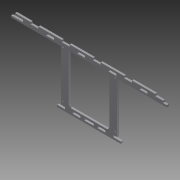
# Autodesk Inventor part: back
Saved by Autodesk Inventor 2011 (Build 150239000, 239)
## iProperties
Created: 2011-08-21
Part Number: back
Document SubType Name: Modeling
Designer: Matthew
Density: 1 g/cm^3
Author: Matthew
Autodesk Inventor part; units mm, degrees
ref_plane "YZ Plane" through (0, 0, 0) normal (1, 0, 0) x (0, 1, 0)
ref_plane "XZ Plane" through (0, 0, 0) normal (0, 1, 0) x (-1, 0, 0)
ref_plane "XY Plane" through (0, 0, 0) normal (0, 0, 1) x (1, 0, 0)
sketch "Sketch1" plane through (0, 0, 0) normal (0, 0, 1) x (1, 0, 0)
  line L0 (-267.7504, 67.4597) -> (240.2496, 67.4597)
  line L1 (240.2496, 67.4597) -> (240.2496, -986.6403)
  line L2 (240.2496, -986.6403) -> (-267.7504, -986.6403)
  line L3 (-267.7504, -986.6403) -> (-267.7504, 67.4597)
  point P0 (0, 0)
  dimension "d0" = 508
  dimension "d1" = 1054.1
  constraints: 8 end point, 2 parallel, 1 horizontal, 1 perpendicular
  measures "d0" distance of L1.end L2.end
  measures "d1" distance of L0.end L1.end
extrude "Extrusion1" add sketch "Sketch1" along normal blind 6.35
sketch "Sketch2" plane through (0, 0, 6.35) normal (0, 0, 1) x (1, 0, 0)
  line L0 (240.2496, -986.6403) -> (-267.7504, -986.6403) projected
  line L1 (-267.7504, -986.6403) -> (-13.7504, -986.6403)
  line L2 (-13.7504, -986.6403) -> (-13.7504, -980.2903)
  line L3 (-13.7504, -980.2903) -> (1.4896, -980.2903)
  line L4 (1.4896, -980.2903) -> (-28.9904, -980.2903)
  line L5 (-28.9904, -980.2903) -> (1.4896, -980.2903)
  line L6 (1.4896, -980.2903) -> (1.4896, -973.9403)
  line L7 (1.4896, -973.9403) -> (-28.9904, -973.9403)
  line L8 (-28.9904, -973.9403) -> (-28.9904, -980.2903)
  point P0 (0, 0)
  dimension "d4" = 254
  dimension "d5" = 6.35
  dimension "d6" = 15.24
  dimension "d7" = 30.48
  dimension "d8" = 6.35
  constraints: 16 end point, 4 parallel, 2 perpendicular, 1 horizontal, 1 midpoint
  measures "d4" distance of L0.end L1.end
  measures "d5" distance of L1.end L2.end
  measures "d6" distance of L2.end L3.end
  measures "d7" distance of L3.end L4.end
  measures "d8" distance of L6.end L5.end
extrude "Extrusion2" cut sketch "Sketch2" against normal blind 104.14
sketch "Sketch3" plane through (0, 0, 6.35) normal (0, 0, 1) x (1, 0, 0)
  line L0 (240.2496, -986.6403) -> (-267.7504, -986.6403) projected
  line L1 (1.4896, -980.2903) -> (14.1896, -980.2903)
  line L2 (-28.9904, -980.2903) -> (-41.6904, -980.2903)
  line L3 (-41.6904, -980.2903) -> (-67.0904, -980.2903)
  line L4 (-67.0904, -980.2903) -> (-67.0904, -973.9403)
  line L5 (-67.0904, -973.9403) -> (-41.6904, -973.9403)
  line L6 (-41.6904, -973.9403) -> (-41.6904, -980.2903)
  line L7 (14.1896, -980.2903) -> (39.5896, -980.2903)
  line L8 (39.5896, -980.2903) -> (39.5896, -973.9403)
  line L9 (39.5896, -973.9403) -> (14.1896, -973.9403)
  line L10 (14.1896, -973.9403) -> (14.1896, -980.2903)
  point P0 (0, 0)
  dimension "d11" = 12.7
  dimension "d12" = 12.7
  dimension "d13" = 25.4
  dimension "d14" = 25.4
  constraints: 20 end point, 5 parallel, 2 horizontal, 2 perpendicular, 1 collinear
  measures "d11" distance of L1.start L1.end
  measures "d12" distance of L2.start L2.end
  measures "d13" distance of L4.end L5.end
  measures "d14" distance of L9.end L8.end
extrude "Extrusion3" cut sketch "Sketch3" against normal blind 104.14
sketch "Sketch4" plane through (0, 0, 6.35) normal (0, 0, 1) x (1, 0, 0)
  line L0 (-67.0904, -973.9403) -> (-41.6904, -973.9403) projected
  line L1 (14.1896, -973.9403) -> (39.5896, -973.9403) projected
  line L2 (-28.9904, -973.9403) -> (1.4896, -973.9403) projected
  line L3 (240.2496, 67.4597) -> (240.2496, -986.6403) projected
  line L4 (-267.7504, -986.6403) -> (-267.7504, 67.4597) projected
  line L5 (240.2496, -986.6403) -> (-267.7504, -986.6403) projected
  line L6 (-67.0904, -980.2903) -> (-92.4904, -980.2903)
  line L7 (-92.4904, -980.2903) -> (-117.8904, -980.2903)
  line L8 (-117.8904, -980.2903) -> (-117.8904, -986.6403)
  line L9 (39.5896, -980.2903) -> (64.9896, -980.2903)
  line L10 (64.9896, -980.2903) -> (90.3896, -980.2903)
  line L11 (90.3896, -980.2903) -> (90.3896, -986.6403)
  line L12 (-41.6904, -973.9403) -> (-28.9904, -973.9403)
  line L13 (1.4896, -973.9403) -> (14.1896, -973.9403)
  line L14 (-67.0904, -973.9403) -> (-79.7904, -973.9403)
  line L15 (39.5896, -973.9403) -> (52.2896, -973.9403)
  line L16 (-79.7904, -973.9403) -> (-79.7904, -802.4903)
  line L17 (52.2896, -973.9403) -> (52.2896, -802.4903)
  line L18 (52.2896, -802.4903) -> (-79.7904, -802.4903)
  line L19 (-79.7904, -802.4903) -> (-105.1904, -802.4903)
  line L20 (-105.1904, -802.4903) -> (-105.1904, -815.1903)
  line L21 (-105.1904, -815.1903) -> (-92.4904, -815.1903)
  line L22 (-92.4904, -815.1903) -> (-92.4904, -980.2903)
  line L23 (64.9896, -980.2903) -> (64.9896, -815.1903)
  line L24 (64.9896, -815.1903) -> (77.6896, -815.1903)
  line L25 (77.6896, -815.1903) -> (77.6896, -802.4903)
  line L26 (77.6896, -802.4903) -> (52.2896, -802.4903)
  line L27 (-105.1904, -802.4903) -> (-267.7504, -802.4903)
  line L28 (77.6896, -802.4903) -> (240.2496, -802.4903)
  point P0 (0, 0)
  dimension "d17" = 25.4
  dimension "d18" = 25.4
  dimension "d19" = 25.4
  dimension "d20" = 25.4
  dimension "d21" = 171.45
  dimension "d22" = 25.4
  dimension "d23" = 12.7
  constraints: 46 end point, 10 perpendicular, 8 parallel, 5 collinear, 4 point on line
  measures "d17" distance of L6.start L6.end
  measures "d18" distance of L6.end L7.end
  measures "d19" distance of L9.start L9.end
  measures "d20" distance of L9.end L10.end
  measures "d21" distance of L14.end L16.end
  measures "d22" distance of L16.end L19.end
  measures "d23" distance of L19.end L20.end
extrude "Extrusion4" cut sketch "Sketch4" against normal blind 104.14 contours L14 L16 L18 L17 L15 L1 L13 L2 L12 L0 | L20 L21 L22 L7 L8 L5 L4 L27 | L28 L3 L5 L11 L10 L23 L24 L25
sketch "Sketch5" plane through (0, 0, 6.35) normal (0, 0, 1) x (1, 0, 0)
  line L0 (-92.4904, -815.1903) -> (-92.4904, -980.2903) projected
  line L1 (64.9896, -980.2903) -> (64.9896, -815.1903) projected
  line L2 (-92.4904, -973.9403) -> (-92.4904, -967.5903)
  line L3 (-92.4904, -967.5903) -> (-105.1904, -967.5903)
  line L4 (-105.1904, -967.5903) -> (-105.1904, -954.8903)
  line L5 (-105.1904, -954.8903) -> (-92.4904, -954.8903)
  line L6 (64.9896, -954.8903) -> (77.6896, -954.8903)
  line L7 (77.6896, -954.8903) -> (77.6896, -967.5903)
  line L8 (77.6896, -967.5903) -> (64.9896, -967.5903)
  point P0 (0, 0)
  dimension "d26" = 6.35
  dimension "d27" = 12.7
  constraints: 14 end point, 5 point on line, 3 perpendicular, 2 parallel, 1 collinear
  measures "d26" distance of L2.start L2.end
  measures "d27" distance of L3.end L4.end
extrude "Extrusion5" add sketch "Sketch5" against normal blind 6.35
sketch "Sketch6" plane through (0, 0, 6.35) normal (0, 0, 1) x (1, 0, 0)
  line L0 (-79.7904, -802.4903) -> (52.2896, -802.4903) projected
  line L1 (-267.7504, -802.4903) -> (-105.1904, -802.4903) projected
  line L2 (77.6896, -802.4903) -> (240.2496, -802.4903) projected
  line L3 (-267.7504, -802.4903) -> (-242.3504, -802.4903)
  line L4 (-242.3504, -802.4903) -> (-216.9504, -802.4903)
  line L5 (-216.9504, -802.4903) -> (-140.7504, -802.4903)
  line L6 (-140.7504, -802.4903) -> (-115.3504, -802.4903)
  line L7 (-115.3504, -802.4903) -> (-39.1504, -802.4903)
  line L8 (-39.1504, -802.4903) -> (-13.7504, -802.4903)
  line L9 (-13.7504, -802.4903) -> (62.4496, -802.4903)
  line L10 (62.4496, -802.4903) -> (87.8496, -802.4903)
  line L11 (87.8496, -802.4903) -> (164.0496, -802.4903)
  line L12 (164.0496, -802.4903) -> (189.4496, -802.4903)
  line L13 (189.4496, -802.4903) -> (265.6496, -802.4903)
  line L14 (265.6496, -802.4903) -> (240.2496, -802.4903)
  line L15 (-242.3504, -802.4903) -> (-216.9504, -802.4903)
  line L16 (-216.9504, -802.4903) -> (-216.9504, -796.1403)
  line L17 (-216.9504, -796.1403) -> (-242.3504, -796.1403)
  line L18 (-242.3504, -796.1403) -> (-242.3504, -802.4903)
  line L19 (-140.7504, -802.4903) -> (-115.3504, -802.4903)
  line L20 (-115.3504, -802.4903) -> (-115.3504, -796.1403)
  line L21 (-115.3504, -796.1403) -> (-140.7504, -796.1403)
  line L22 (-140.7504, -796.1403) -> (-140.7504, -802.4903)
  line L23 (-39.1504, -802.4903) -> (-13.7504, -802.4903)
  line L24 (-13.7504, -802.4903) -> (-13.7504, -796.1403)
  line L25 (-13.7504, -796.1403) -> (-39.1504, -796.1403)
  line L26 (-39.1504, -796.1403) -> (-39.1504, -802.4903)
  line L27 (62.4496, -802.4903) -> (87.8496, -802.4903)
  line L28 (87.8496, -802.4903) -> (87.8496, -796.1403)
  line L29 (87.8496, -796.1403) -> (62.4496, -796.1403)
  line L30 (62.4496, -796.1403) -> (62.4496, -802.4903)
  line L31 (164.0496, -802.4903) -> (189.4496, -802.4903)
  line L32 (189.4496, -802.4903) -> (189.4496, -796.1403)
  line L33 (189.4496, -796.1403) -> (164.0496, -796.1403)
  line L34 (164.0496, -796.1403) -> (164.0496, -802.4903)
  point P0 (0, 0)
  dimension "d30" = 25.4
  dimension "d31" = 25.4
  dimension "d32" = 76.2
  dimension "d33" = 25.4
  dimension "d34" = 76.2
  dimension "d35" = 25.4
  dimension "d36" = 76.2
  dimension "d37" = 25.4
  dimension "d38" = 76.2
  dimension "d39" = 25.4
  dimension "d40" = 76.2
  dimension "d41" = 25.4
  dimension "d42" = 6.35
  constraints: 64 end point, 10 parallel, 10 point on line, 5 horizontal, 5 perpendicular, 1 collinear, 1 midpoint
  measures "d30" distance of L1.start L3.end
  measures "d31" distance of L3.end L4.end
  measures "d32" distance of L4.end L5.end
  measures "d33" distance of L5.end L6.end
  measures "d34" distance of L6.end L7.end
  measures "d35" distance of L7.end L8.end
  measures "d36" distance of L8.end L9.end
  measures "d37" distance of L9.end L10.end
  measures "d38" distance of L10.end L11.end
  measures "d39" distance of L11.end L12.end
  measures "d40" distance of L12.end L13.end
  measures "d41" distance of L13.end L2.end
  measures "d42" distance of L16.end L15.end
extrude "Extrusion6" cut sketch "Sketch6" against normal blind 25.4
sketch "Sketch7" plane through (0, 0, 6.35) normal (0, 0, 1) x (1, 0, 0)
  line L0 (-267.7504, -802.4903) -> (240.2496, -802.4903)
  line L1 (240.2496, -802.4903) -> (240.2496, -808.8403)
  line L2 (240.2496, -808.8403) -> (-267.7504, -808.8403)
  line L3 (-267.7504, -808.8403) -> (-267.7504, -802.4903)
  point P0 (0, 0)
  constraints: 8 end point, 2 parallel, 1 horizontal, 1 perpendicular
extrude "Extrusion7" add sketch "Sketch7" against normal blind 6.35
sketch "Sketch8" plane through (0, 0, 6.35) normal (0, 0, 1) x (1, 0, 0)
  line L0 (-216.9504, -796.1403) -> (-191.5504, -796.1403)
  line L1 (-191.5504, -796.1403) -> (-191.5504, -789.7903)
  line L2 (-191.5504, -789.7903) -> (-216.9504, -789.7903)
  line L3 (-216.9504, -789.7903) -> (-216.9504, -796.1403)
  line L4 (-115.3504, -796.1403) -> (-89.9504, -796.1403)
  line L5 (-89.9504, -796.1403) -> (-89.9504, -789.7903)
  line L6 (-89.9504, -789.7903) -> (-115.3504, -789.7903)
  line L7 (-115.3504, -789.7903) -> (-115.3504, -796.1403)
  line L8 (-13.7504, -796.1403) -> (11.6496, -796.1403)
  line L9 (11.6496, -796.1403) -> (11.6496, -789.7903)
  line L10 (11.6496, -789.7903) -> (-13.7504, -789.7903)
  line L11 (-13.7504, -789.7903) -> (-13.7504, -796.1403)
  line L12 (87.8496, -796.1403) -> (113.2496, -796.1403)
  line L13 (113.2496, -796.1403) -> (113.2496, -789.7903)
  line L14 (113.2496, -789.7903) -> (87.8496, -789.7903)
  line L15 (87.8496, -789.7903) -> (87.8496, -796.1403)
  line L16 (189.4496, -796.1403) -> (214.8496, -796.1403)
  line L17 (214.8496, -796.1403) -> (214.8496, -789.7903)
  line L18 (214.8496, -789.7903) -> (189.4496, -789.7903)
  line L19 (189.4496, -789.7903) -> (189.4496, -796.1403)
  point P0 (0, 0)
  dimension "d47" = 25.4
  dimension "d48" = 6.35
  dimension "d49" = 25.4
  dimension "d50" = 25.4
  dimension "d51" = 25.4
  dimension "d52" = 25.4
  constraints: 40 end point, 10 parallel, 5 horizontal, 5 perpendicular
  measures "d47" distance of L2.end L1.end
  measures "d48" distance of L1.end L0.end
  measures "d49" distance of L6.end L5.end
  measures "d50" distance of L10.end L9.end
  measures "d51" distance of L14.end L13.end
  measures "d52" distance of L18.end L17.end
extrude "Extrusion8" cut sketch "Sketch8" against normal blind 6.35
sketch "Sketch9" plane through (0, 0, 6.35) normal (0, 0, 1) x (1, 0, 0)
  circle A0 centre (-98.8404, -808.8403) radius 1.9812
  circle A1 centre (-98.8404, -961.2403) radius 1.9812
  circle A2 centre (71.3396, -961.2403) radius 1.9812
  circle A3 centre (71.3396, -808.8403) radius 1.9812
  point P0 (0, 0)
  dimension "d55" = 3.9624
  dimension "d56" = 3.9624
  dimension "d57" = 3.9624
  dimension "d58" = 3.9624
  constraints: 4 centre point
  measures "d55" diameter of A0
  measures "d56" diameter of A1
  measures "d57" diameter of A2
  measures "d58" diameter of A3
extrude "Extrusion9" cut sketch "Sketch9" against normal blind 6.35
sketch "Sketch10" plane through (0, 0, 0) normal (0, 0, -1) x (-1, 0, 0)
  line L0 (-77.6896, -815.1903) -> (-64.9896, -815.1903) projected
  line L1 (-64.9896, -815.1903) -> (-64.9896, -954.8903) projected
  line L2 (-77.6896, -954.8903) -> (-64.9896, -954.8903) projected
  line L3 (-64.9896, -967.5903) -> (-77.6896, -967.5903) projected
  line L4 (-64.9896, -967.5903) -> (-64.9896, -980.2903) projected
  line L5 (92.4904, -980.2903) -> (92.4904, -967.5903) projected
  line L6 (105.1904, -967.5903) -> (92.4904, -967.5903) projected
  line L7 (92.4904, -954.8903) -> (105.1904, -954.8903) projected
  line L8 (92.4904, -954.8903) -> (92.4904, -815.1903) projected
  line L9 (92.4904, -815.1903) -> (105.1904, -815.1903) projected
  line L10 (-77.6896, -808.8403) -> (-240.2496, -808.8403) projected
  line L11 (-77.6896, -815.1903) -> (-77.6896, -954.8903)
  line L12 (105.1904, -954.8903) -> (105.1904, -815.1903)
  line L13 (105.1904, -967.5903) -> (105.1904, -973.9403)
  line L14 (105.1904, -973.9403) -> (92.4904, -973.9403)
  line L15 (-77.6896, -967.5903) -> (-77.6896, -973.9403)
  line L16 (-77.6896, -973.9403) -> (-64.9896, -973.9403)
  point P0 (0, 0)
  constraints: 12 end point, 2 midpoint, 2 perpendicular, 1 collinear, 1 parallel
extrude "Extrusion10" add sketch "Sketch10" against normal blind 6.35
sketch "Sketch11" plane through (0, 0, 0) normal (0, 0, -1) x (-1, 0, 0)
  line L0 (79.7904, -808.8403) -> (79.7904, -973.9403) projected
  line L1 (79.7904, -973.9403) -> (67.0904, -973.9403) projected
  line L2 (-39.5896, -973.9403) -> (-52.2896, -973.9403) projected
  line L3 (-52.2896, -973.9403) -> (-52.2896, -808.8403) projected
  line L4 (-39.5896, -973.9403) -> (-52.2896, -961.2403)
  line L5 (67.0904, -973.9403) -> (79.7904, -961.2403)
  line L6 (-45.9396, -967.5903) -> (73.4404, -967.5903)
  line L7 (-39.5896, -973.9403) -> (67.0904, -973.9403)
  point P0 (0, 0)
  constraints: 8 end point, 2 midpoint, 2 point on line, 1 perpendicular
extrude "Extrusion11" add sketch "Sketch11" against normal blind 6.35
sketch "Sketch12" plane through (0, 0, 0) normal (0, 0, -1) x (-1, 0, 0)
  line L0 (267.7504, -808.8403) -> (267.7504, 67.4597) projected
  line L1 (-240.2496, 67.4597) -> (-240.2496, -808.8403) projected
  line L2 (-240.2496, 67.4597) -> (-214.8496, 67.4597)
  line L3 (-214.8496, 67.4597) -> (-214.8496, 42.0597)
  line L4 (-214.8496, 42.0597) -> (-240.2496, 42.0597)
  line L5 (-240.2496, 42.0597) -> (-240.2496, 67.4597)
  line L6 (267.7504, 67.4597) -> (242.3504, 67.4597)
  line L7 (242.3504, 67.4597) -> (242.3504, 42.0597)
  line L8 (242.3504, 42.0597) -> (267.7504, 42.0597)
  line L9 (267.7504, 42.0597) -> (267.7504, 67.4597)
  line L10 (-240.2496, -789.7903) -> (-214.8496, -789.7903)
  line L11 (-214.8496, -789.7903) -> (-214.8496, -764.3903)
  line L12 (-214.8496, -764.3903) -> (-240.2496, -764.3903)
  line L13 (-240.2496, -764.3903) -> (-240.2496, -789.7903)
  line L14 (267.7504, -789.7903) -> (242.3504, -789.7903)
  line L15 (242.3504, -789.7903) -> (242.3504, -764.3903)
  line L16 (242.3504, -764.3903) -> (267.7504, -764.3903)
  line L17 (267.7504, -764.3903) -> (267.7504, -789.7903)
  line L18 (-214.8496, -764.3903) -> (242.3504, -764.3903)
  line L19 (242.3504, -764.3903) -> (242.3504, 42.0597)
  line L20 (242.3504, 42.0597) -> (-214.8496, 42.0597)
  line L21 (-214.8496, 42.0597) -> (-214.8496, -764.3903)
  point P0 (0, 0)
  dimension "d65" = 25.4
  dimension "d66" = 25.4
  dimension "d67" = 25.4
  dimension "d68" = 25.4
  dimension "d69" = 25.4
  dimension "d70" = 25.4
  dimension "d71" = 25.4
  dimension "d72" = 25.4
  constraints: 40 end point, 10 parallel, 5 horizontal, 5 perpendicular, 2 point on line
  measures "d65" distance of L3.end L4.end
  measures "d66" distance of L2.end L3.end
  measures "d67" distance of L8.end L7.end
  measures "d68" distance of L7.end L6.end
  measures "d69" distance of L12.end L11.end
  measures "d70" distance of L11.end L10.end
  measures "d71" distance of L15.end L16.end
  measures "d72" distance of L14.end L15.end
extrude "Extrusion12" cut sketch "Sketch12" against normal blind 6.35 contours L18 L21 L20 L19
fillet "Fillet1" radius 12.7 1 edges at (-242.3504, 42.0597, 3.175)
fillet "Fillet2" radius 12.7 3 edges at (214.8496, 42.0597, 3.175) (214.8496, -764.3903, 3.175) (-242.3504, -764.3903, 3.175)
sketch "Sketch13" plane through (0, 0, 0) normal (0, 0, -1) x (-1, 0, 0)
  line L0 (-214.8496, -751.6903) -> (-214.8496, 29.3597) projected
  arc A0 (-202.1496, 42.0597) -> (-214.8496, 29.3597) centre (-202.1496, 29.3597) ccw projected
  line L1 (-202.1496, 42.0597) -> (229.6504, 42.0597) projected
  arc A1 (242.3504, 29.3597) -> (229.6504, 42.0597) centre (229.6504, 29.3597) ccw projected
  line L2 (242.3504, 29.3597) -> (242.3504, -751.6903) projected
  arc A2 (229.6504, -764.3903) -> (242.3504, -751.6903) centre (229.6504, -751.6903) ccw projected
  arc A3 (-214.8496, -751.6903) -> (-202.1496, -764.3903) centre (-202.1496, -751.6903) ccw projected
  line L3 (267.7504, -808.8403) -> (267.7504, 67.4597) projected
  line L4 (267.7504, 67.4597) -> (-240.2496, 67.4597) projected
  line L5 (-240.2496, 67.4597) -> (-240.2496, -808.8403) projected
  line L6 (-202.1496, -764.3903) -> (-240.2496, -764.3903)
  line L7 (229.6504, -764.3903) -> (267.7504, -764.3903)
  point P0 (0, 0)
  constraints: 4 end point, 2 perpendicular, 2 point on line, 2 tangent
extrude "Extrusion13" cut sketch "Sketch13" against normal blind 25.4
sketch "Sketch14" plane through (0, 0, 0) normal (0, 0, -1) x (-1, 0, 0)
  line L0 (-240.2496, -764.3903) -> (-202.1496, -764.3903)
  line L1 (-202.1496, -764.3903) -> (-202.1496, -688.1903)
  line L2 (-202.1496, -688.1903) -> (-240.2496, -688.1903)
  line L3 (-240.2496, -688.1903) -> (-240.2496, -764.3903)
  line L4 (267.7504, -764.3903) -> (229.6504, -764.3903)
  line L5 (229.6504, -764.3903) -> (229.6504, -688.1903)
  line L6 (229.6504, -688.1903) -> (267.7504, -688.1903)
  line L7 (267.7504, -688.1903) -> (267.7504, -764.3903)
  point P0 (0, 0)
  dimension "d79" = 76.2
  dimension "d80" = 76.2
  constraints: 16 end point, 4 parallel, 2 horizontal, 2 perpendicular
  measures "d79" distance of L1.end L0.end
  measures "d80" distance of L4.end L5.end
extrude "Extrusion14" add sketch "Sketch14" against normal blind 6.35
sketch "Sketch15" plane through (0, 0, 0) normal (0, 0, -1) x (-1, 0, 0)
  line L0 (-240.2496, -688.1903) -> (-221.1996, -688.1903)
  line L1 (-221.1996, -688.1903) -> (-221.1996, -707.2403)
  line L2 (-221.1996, -707.2403) -> (-240.2496, -707.2403)
  line L3 (-240.2496, -707.2403) -> (-240.2496, -688.1903)
  line L4 (267.7504, -688.1903) -> (248.7004, -688.1903)
  line L5 (248.7004, -688.1903) -> (248.7004, -707.2403)
  line L6 (248.7004, -707.2403) -> (267.7504, -707.2403)
  line L7 (267.7504, -707.2403) -> (267.7504, -688.1903)
  circle A0 centre (248.7004, -707.2403) radius 1.9812
  circle A1 centre (-221.1996, -707.2403) radius 1.9812
  point P0 (0, 0)
  dimension "d83" = 19.05
  dimension "d84" = 19.05
  dimension "d85" = 19.05
  dimension "d86" = 19.05
  dimension "d87" = 3.9624
  dimension "d88" = 3.9624
  constraints: 16 end point, 4 parallel, 2 centre point, 2 coincident, 2 horizontal, 2 perpendicular
  measures "d83" distance of L1.end L2.end
  measures "d84" distance of L0.end L1.end
  measures "d85" distance of L6.end L5.end
  measures "d86" distance of L5.end L4.end
  measures "d87" diameter of A0
  measures "d88" diameter of A1
extrude "Extrusion15" cut sketch "Sketch15" against normal blind 6.35 contours A1 L2 L1 | L1 L2 A1 | A0 L6 L5 | L5 L6 A0
sketch "Sketch16" plane through (0, 0, 0) normal (0, 0, -1) x (-1, 0, 0)
  line L0 (-240.2496, -688.1903) -> (-240.2496, -808.8403) projected
  line L1 (-240.2496, -688.1903) -> (-233.8996, -688.1903)
  line L2 (-233.8996, -688.1903) -> (-233.8996, -713.5903)
  line L3 (-233.8996, -713.5903) -> (-240.2496, -713.5903)
  line L4 (-240.2496, -713.5903) -> (-240.2496, -688.1903)
  line L5 (-233.8996, -713.5903) -> (-240.2496, -713.5903)
  line L6 (-240.2496, -713.5903) -> (-240.2496, -738.9903)
  line L7 (-240.2496, -738.9903) -> (-233.8996, -738.9903)
  line L8 (-233.8996, -738.9903) -> (-233.8996, -713.5903)
  line L9 (-233.8996, -738.9903) -> (-240.2496, -738.9903)
  line L10 (-240.2496, -738.9903) -> (-240.2496, -764.3903)
  line L11 (-240.2496, -764.3903) -> (-233.8996, -764.3903)
  line L12 (-233.8996, -764.3903) -> (-233.8996, -738.9903)
  line L13 (-233.8996, -764.3903) -> (-240.2496, -764.3903)
  line L14 (-240.2496, -764.3903) -> (-240.2496, -789.7903)
  line L15 (-240.2496, -789.7903) -> (-233.8996, -789.7903)
  line L16 (-233.8996, -789.7903) -> (-233.8996, -764.3903)
  point P0 (0, 0)
  dimension "d91" = 6.35
  dimension "d92" = 25.4
  dimension "d93" = 25.4
  dimension "d94" = 25.4
  constraints: 32 end point, 8 parallel, 4 horizontal, 4 perpendicular, 3 point on line
  measures "d91" distance of L2.end L3.end
  measures "d92" distance of L1.end L2.end
  measures "d93" distance of L6.end L5.end
  measures "d94" distance of L10.end L9.end
extrude "Extrusion16" cut sketch "Sketch16" against normal blind 6.35 contours L1 L2 L3 L0 | L7 L12 L11 L0
sketch "Sketch17" plane through (0, 0, 0) normal (0, 0, -1) x (-1, 0, 0)
  line L0 (267.7504, -808.8403) -> (267.7504, -688.1903) projected
  line L1 (267.7504, -688.1903) -> (261.4004, -688.1903)
  line L2 (261.4004, -688.1903) -> (261.4004, -713.5903)
  line L3 (261.4004, -713.5903) -> (267.7504, -713.5903)
  line L4 (267.7504, -713.5903) -> (267.7504, -688.1903)
  line L5 (261.4004, -713.5903) -> (267.7504, -713.5903)
  line L6 (267.7504, -713.5903) -> (267.7504, -738.9903)
  line L7 (267.7504, -738.9903) -> (261.4004, -738.9903)
  line L8 (261.4004, -738.9903) -> (261.4004, -713.5903)
  line L9 (261.4004, -738.9903) -> (267.7504, -738.9903)
  line L10 (267.7504, -738.9903) -> (267.7504, -764.3903)
  line L11 (267.7504, -764.3903) -> (261.4004, -764.3903)
  line L12 (261.4004, -764.3903) -> (261.4004, -738.9903)
  point P0 (0, 0)
  dimension "d97" = 6.35
  dimension "d98" = 25.4
  dimension "d99" = 25.4
  dimension "d100" = 25.4
  constraints: 24 end point, 6 parallel, 3 horizontal, 3 perpendicular, 2 point on line
  measures "d97" distance of L3.end L2.end
  measures "d98" distance of L2.end L1.end
  measures "d99" distance of L5.end L6.end
  measures "d100" distance of L9.end L10.end
extrude "Extrusion17" cut sketch "Sketch17" against normal blind 6.35 contours L11 L12 L7 L0 | L3 L2 L1 L0
sketch "Sketch18" plane through (0, 0, 0) normal (0, 0, -1) x (-1, 0, 0)
  circle A0 centre (-221.1996, -707.2403) radius 1.9812 projected
  circle A1 centre (248.7004, -707.2403) radius 1.9812 projected
  line L0 (-233.8996, -688.1903) -> (261.4004, -688.1903)
  line L1 (261.4004, -688.1903) -> (261.4004, -713.5903)
  line L2 (261.4004, -713.5903) -> (-233.8996, -713.5903)
  line L3 (-233.8996, -713.5903) -> (-233.8996, -688.1903)
  point P0 (0, 0)
  constraints: 8 end point, 2 parallel, 1 horizontal, 1 perpendicular
extrude "Extrusion18" cut sketch "Sketch18" against normal blind 25.4
sketch "Sketch19" plane through (0, 0, 0) normal (0, 0, -1) x (-1, 0, 0)
  line L0 (-202.1496, -713.5903) -> (-221.1996, -713.5903)
  line L1 (-221.1996, -713.5903) -> (-221.1996, -726.2903)
  line L2 (-221.1996, -726.2903) -> (-202.1496, -726.2903)
  line L3 (-202.1496, -726.2903) -> (-202.1496, -713.5903)
  circle A0 centre (-221.1996, -726.2903) radius 1.9812
  circle A1 centre (248.7004, -728.2715) radius 1.9812
  point P0 (0, 0)
  dimension "d105" = 19.05
  dimension "d106" = 12.7
  dimension "d107" = 3.9624
  dimension "d108" = 3.9624
  constraints: 8 end point, 2 centre point, 2 parallel, 1 coincident, 1 horizontal, 1 perpendicular
  measures "d105" distance of L2.end L1.end
  measures "d106" distance of L1.end L0.end
  measures "d107" diameter of A0
  measures "d108" diameter of A1
extrude "Extrusion19" cut sketch "Sketch19" against normal blind 25.4 contours A0 L2 L1 | L1 L2 A0 | A1
sketch "Sketch20" plane through (0, 0, 0) normal (0, 0, -1) x (-1, 0, 0)
  line L0 (-214.8496, -789.7903) -> (242.3504, -789.7903)
  line L1 (242.3504, -789.7903) -> (242.3504, -802.4903)
  line L2 (242.3504, -802.4903) -> (-214.8496, -802.4903)
  line L3 (-214.8496, -802.4903) -> (-214.8496, -789.7903)
  point P0 (0, 0)
  constraints: 8 end point, 2 parallel, 1 horizontal, 1 perpendicular
extrude "Extrusion20" add sketch "Sketch20" against normal blind 6.35
sketch "Sketch21" plane through (0, 0, 0) normal (0, 0, -1) x (-1, 0, 0)
  line L0 (-240.2496, -808.8403) -> (-227.5496, -808.8403)
  line L1 (-227.5496, -808.8403) -> (-227.5496, -796.1403)
  line L2 (-227.5496, -796.1403) -> (-240.2496, -796.1403)
  line L3 (-240.2496, -796.1403) -> (-240.2496, -808.8403)
  line L4 (-227.5496, -796.1403) -> (-202.1496, -796.1403)
  line L5 (-202.1496, -796.1403) -> (-202.1496, -789.7903)
  line L6 (-202.1496, -789.7903) -> (-227.5496, -789.7903)
  line L7 (-227.5496, -789.7903) -> (-227.5496, -796.1403)
  line L8 (-202.1496, -796.1403) -> (-176.7496, -796.1403)
  line L9 (-176.7496, -796.1403) -> (-176.7496, -802.4903)
  line L10 (-176.7496, -802.4903) -> (-202.1496, -802.4903)
  line L11 (-202.1496, -802.4903) -> (-202.1496, -796.1403)
  line L12 (-176.7496, -796.1403) -> (-151.3496, -796.1403)
  line L13 (-151.3496, -796.1403) -> (-151.3496, -802.4903)
  line L14 (-151.3496, -802.4903) -> (-176.7496, -802.4903)
  line L15 (-176.7496, -802.4903) -> (-176.7496, -796.1403)
  line L16 (-151.3496, -796.1403) -> (-125.9496, -796.1403)
  line L17 (-125.9496, -796.1403) -> (-125.9496, -802.4903)
  line L18 (-125.9496, -802.4903) -> (-151.3496, -802.4903)
  line L19 (-151.3496, -802.4903) -> (-151.3496, -796.1403)
  line L20 (-125.9496, -796.1403) -> (-100.5496, -796.1403)
  line L21 (-100.5496, -796.1403) -> (-100.5496, -789.7903)
  line L22 (-100.5496, -789.7903) -> (-125.9496, -789.7903)
  line L23 (-125.9496, -789.7903) -> (-125.9496, -796.1403)
  line L24 (-100.5496, -796.1403) -> (-75.1496, -796.1403)
  line L25 (-75.1496, -796.1403) -> (-75.1496, -802.4903)
  line L26 (-75.1496, -802.4903) -> (-100.5496, -802.4903)
  line L27 (-100.5496, -802.4903) -> (-100.5496, -796.1403)
  line L28 (-75.1496, -802.4903) -> (-49.7496, -802.4903)
  line L29 (-49.7496, -802.4903) -> (-49.7496, -796.1403)
  line L30 (-49.7496, -796.1403) -> (-75.1496, -796.1403)
  line L31 (-75.1496, -796.1403) -> (-75.1496, -802.4903)
  line L32 (-49.7496, -796.1403) -> (-24.3496, -796.1403)
  line L33 (-24.3496, -796.1403) -> (-24.3496, -802.4903)
  line L34 (-24.3496, -802.4903) -> (-49.7496, -802.4903)
  line L35 (-49.7496, -802.4903) -> (-49.7496, -796.1403)
  line L36 (-24.3496, -796.1403) -> (1.0504, -796.1403)
  line L37 (1.0504, -796.1403) -> (1.0504, -789.7903)
  line L38 (1.0504, -789.7903) -> (-24.3496, -789.7903)
  line L39 (-24.3496, -789.7903) -> (-24.3496, -796.1403)
  line L40 (1.0504, -796.1403) -> (26.4504, -796.1403)
  line L41 (26.4504, -796.1403) -> (26.4504, -802.4903)
  line L42 (26.4504, -802.4903) -> (1.0504, -802.4903)
  line L43 (1.0504, -802.4903) -> (1.0504, -796.1403)
  line L44 (26.4504, -796.1403) -> (51.8504, -796.1403)
  line L45 (51.8504, -796.1403) -> (51.8504, -802.4903)
  line L46 (51.8504, -802.4903) -> (26.4504, -802.4903)
  line L47 (26.4504, -802.4903) -> (26.4504, -796.1403)
  line L48 (51.8504, -796.1403) -> (77.2504, -796.1403)
  line L49 (77.2504, -796.1403) -> (77.2504, -802.4903)
  line L50 (77.2504, -802.4903) -> (51.8504, -802.4903)
  line L51 (51.8504, -802.4903) -> (51.8504, -796.1403)
  line L52 (77.2504, -796.1403) -> (102.6504, -796.1403)
  line L53 (102.6504, -796.1403) -> (102.6504, -789.7903)
  line L54 (102.6504, -789.7903) -> (77.2504, -789.7903)
  line L55 (77.2504, -789.7903) -> (77.2504, -796.1403)
  line L56 (102.6504, -796.1403) -> (128.0504, -796.1403)
  line L57 (128.0504, -796.1403) -> (128.0504, -802.4903)
  line L58 (128.0504, -802.4903) -> (102.6504, -802.4903)
  line L59 (102.6504, -802.4903) -> (102.6504, -796.1403)
  line L60 (128.0504, -796.1403) -> (153.4504, -796.1403)
  line L61 (153.4504, -796.1403) -> (153.4504, -802.4903)
  line L62 (153.4504, -802.4903) -> (128.0504, -802.4903)
  line L63 (128.0504, -802.4903) -> (128.0504, -796.1403)
  line L64 (153.4504, -796.1403) -> (178.8504, -796.1403)
  line L65 (178.8504, -796.1403) -> (178.8504, -802.4903)
  line L66 (178.8504, -802.4903) -> (153.4504, -802.4903)
  line L67 (153.4504, -802.4903) -> (153.4504, -796.1403)
  line L68 (178.8504, -796.1403) -> (204.2504, -796.1403)
  line L69 (204.2504, -796.1403) -> (204.2504, -789.7903)
  line L70 (204.2504, -789.7903) -> (178.8504, -789.7903)
  line L71 (178.8504, -789.7903) -> (178.8504, -796.1403)
  line L72 (204.2504, -796.1403) -> (229.6504, -796.1403)
  line L73 (229.6504, -796.1403) -> (229.6504, -802.4903)
  line L74 (229.6504, -802.4903) -> (204.2504, -802.4903)
  line L75 (204.2504, -802.4903) -> (204.2504, -796.1403)
  line L76 (229.6504, -796.1403) -> (255.0504, -796.1403)
  line L77 (255.0504, -796.1403) -> (255.0504, -802.4903)
  line L78 (255.0504, -802.4903) -> (229.6504, -802.4903)
  line L79 (229.6504, -802.4903) -> (229.6504, -796.1403)
  point P0 (0, 0)
  dimension "d113" = 12.7
  dimension "d114" = 12.7
  dimension "d115" = 25.4
  dimension "d116" = 6.35
  dimension "d117" = 25.4
  dimension "d118" = 25.4
  dimension "d119" = 25.4
  dimension "d120" = 25.4
  dimension "d121" = 25.4
  dimension "d122" = 25.4
  dimension "d123" = 25.4
  dimension "d124" = 25.4
  dimension "d125" = 25.4
  dimension "d126" = 25.4
  dimension "d127" = 25.4
  dimension "d128" = 25.4
  dimension "d129" = 25.4
  dimension "d130" = 25.4
  dimension "d131" = 25.4
  dimension "d132" = 25.4
  dimension "d133" = 25.4
  dimension "d134" = 25.4
  constraints: 160 end point, 40 parallel, 20 horizontal, 20 perpendicular, 3 point on line
  measures "d113" distance of L2.end L1.end
  measures "d114" distance of L1.end L0.end
  measures "d115" distance of L6.end L5.end
  measures "d116" distance of L5.end L4.end
  measures "d117" distance of L9.end L10.end
  measures "d118" distance of L13.end L14.end
  measures "d119" distance of L17.end L18.end
  measures "d120" distance of L22.end L21.end
  measures "d121" distance of L25.end L26.end
  measures "d122" distance of L30.end L29.end
  measures "d123" distance of L33.end L34.end
  measures "d124" distance of L38.end L37.end
  measures "d125" distance of L41.end L42.end
  measures "d126" distance of L45.end L46.end
  measures "d127" distance of L49.end L50.end
  measures "d128" distance of L54.end L53.end
  measures "d129" distance of L57.end L58.end
  measures "d130" distance of L61.end L62.end
  measures "d131" distance of L65.end L66.end
  measures "d132" distance of L70.end L69.end
  measures "d133" distance of L73.end L74.end
  measures "d134" distance of L77.end L78.end
extrude "Extrusion21" cut sketch "Sketch21" against normal blind 6.35 contours L71 L70 L69 L68 | L55 L54 L53 L52 | L39 L38 L37 L36 | L23 L22 L21 L20 | L7 L6 L5 L4 | L12 L13 L14 L9 | L30 L29 L28 L25 | L44 L45 L46 L41 | L60 L61 L62 L57 | L76 L77 L78 L73
sketch "Sketch22" plane through (0, 0, 0) normal (0, 0, -1) x (-1, 0, 0)
  line L0 (-240.2496, -764.3903) -> (-240.2496, -808.8403) projected
  line L1 (267.7504, -808.8403) -> (267.7504, -764.3903) projected
  line L2 (-227.5496, -789.7903) -> (-240.2496, -789.7903)
  line L3 (-240.2496, -789.7903) -> (-240.2496, -802.4903)
  line L4 (-240.2496, -802.4903) -> (-227.5496, -802.4903)
  line L5 (-227.5496, -802.4903) -> (-227.5496, -789.7903)
  line L6 (255.0504, -802.4903) -> (267.7504, -802.4903)
  line L7 (267.7504, -802.4903) -> (267.7504, -789.7903)
  line L8 (267.7504, -789.7903) -> (255.0504, -789.7903)
  line L9 (255.0504, -789.7903) -> (255.0504, -802.4903)
  point P0 (0, 0)
  constraints: 16 end point, 4 parallel, 2 horizontal, 2 perpendicular, 2 point on line
extrude "Extrusion22" cut sketch "Sketch22" against normal blind 6.35
sketch "Sketch23" plane through (0, 0, 0) normal (0, 0, -1) x (-1, 0, 0)
  circle A0 centre (-221.1996, -726.2903) radius 1.9812 projected
  circle A1 centre (248.7004, -728.2715) radius 1.9812 projected
  line L0 (255.0504, -789.7903) -> (267.7504, -789.7903) projected
  line L1 (267.7504, -789.7903) -> (267.7504, -764.3903) projected
  line L2 (267.7504, -764.3903) -> (261.4004, -764.3903) projected
  line L3 (261.4004, -764.3903) -> (261.4004, -738.9903) projected
  line L4 (261.4004, -738.9903) -> (267.7504, -738.9903) projected
  line L5 (267.7504, -738.9903) -> (267.7504, -713.5903) projected
  line L6 (267.7504, -713.5903) -> (229.6504, -713.5903) projected
  line L7 (229.6504, -713.5903) -> (229.6504, -764.3903) projected
  line L8 (229.6504, -764.3903) -> (-202.1496, -764.3903) projected
  line L9 (-202.1496, -764.3903) -> (-202.1496, -713.5903) projected
  line L10 (-202.1496, -713.5903) -> (-240.2496, -713.5903) projected
  line L11 (-240.2496, -713.5903) -> (-240.2496, -738.9903) projected
  line L12 (-240.2496, -738.9903) -> (-233.8996, -738.9903) projected
  line L13 (-233.8996, -738.9903) -> (-233.8996, -764.3903) projected
  line L14 (-233.8996, -764.3903) -> (-240.2496, -764.3903) projected
  line L15 (-240.2496, -764.3903) -> (-240.2496, -789.7903) projected
  line L16 (-240.2496, -789.7903) -> (-202.1496, -789.7903) projected
  line L17 (-75.1496, -796.1403) -> (-49.7496, -796.1403) projected
  line L18 (-202.1496, -789.7903) -> (255.0504, -789.7903)
  point P0 (0, 0)
  constraints: 2 end point, 1 parallel
extrude "Extrusion23" cut sketch "Sketch23" against normal blind 25.4
body "Solid1"
